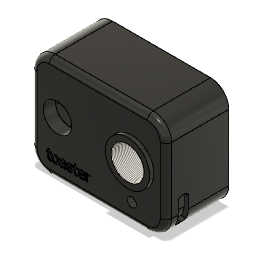
MDCEnclosure (Autodesk Fusion 360 design; units mm, degrees)
Autodesk Fusion 360 part; units mm, degrees
sketch "Board" plane through (0, 0, 0) normal (0, 0, 1) x (1, 0, 0)
  line L0 (4.75, 0) -> (39.105, 0)
  line L1 (43.855, 4.75) -> (43.855, 27.9)
  line L2 (39.105, 32.65) -> (4.75, 32.65)
  line L3 (0, 27.9) -> (0, 4.75)
  arc A0 (4.75, 32.65) -> (0, 27.9) centre (4.75, 27.9) ccw
  arc A1 (43.855, 27.9) -> (39.105, 32.65) centre (39.105, 27.9) ccw
  arc A2 (39.105, 0) -> (43.855, 4.75) centre (39.105, 4.75) ccw
  arc A3 (0, 4.75) -> (4.75, 0) centre (4.75, 4.75) ccw
  line L4 (-0.15, 27.9) -> (-0.15, 4.75)
  arc A4 (-0.15, 4.75) -> (4.75, -0.15) centre (4.75, 4.75) ccw
  line L5 (4.75, -0.15) -> (39.105, -0.15)
  arc A5 (39.105, -0.15) -> (44.005, 4.75) centre (39.105, 4.75) ccw
  line L6 (44.005, 4.75) -> (44.005, 27.9)
  arc A6 (44.005, 27.9) -> (39.105, 32.8) centre (39.105, 27.9) ccw
  line L7 (39.105, 32.8) -> (4.75, 32.8)
  arc A7 (4.75, 32.8) -> (-0.15, 27.9) centre (4.75, 27.9) ccw
  line L8 (-0.35, 27.9) -> (-0.35, 4.75)
  arc A8 (-0.35, 4.75) -> (4.75, -0.35) centre (4.75, 4.75) ccw
  line L9 (4.75, -0.35) -> (39.105, -0.35)
  arc A9 (39.105, -0.35) -> (44.205, 4.75) centre (39.105, 4.75) ccw
  line L10 (44.205, 4.75) -> (44.205, 27.9)
  arc A10 (44.205, 27.9) -> (39.105, 33) centre (39.105, 27.9) ccw
  line L11 (39.105, 33) -> (4.75, 33)
  arc A11 (4.75, 33) -> (-0.35, 27.9) centre (4.75, 27.9) ccw
  line L12 (-0.425, 27.9) -> (-0.425, 4.75)
  arc A12 (-0.425, 4.75) -> (4.75, -0.425) centre (4.75, 4.75) ccw
  line L13 (4.75, -0.425) -> (39.105, -0.425)
  arc A13 (39.105, -0.425) -> (44.28, 4.75) centre (39.105, 4.75) ccw
  line L14 (44.28, 4.75) -> (44.28, 27.9)
  arc A14 (44.28, 27.9) -> (39.105, 33.075) centre (39.105, 27.9) ccw
  line L15 (39.105, 33.075) -> (4.75, 33.075)
  arc A15 (4.75, 33.075) -> (-0.425, 27.9) centre (4.75, 27.9) ccw
  line L16 (21.9275, 32.65) -> (21.9275, 0)
  line L17 (21.9275, 33.075) -> (-21.9275, 33.075)
  line L18 (-21.9275, 33.075) -> (-21.9275, -0.425)
  line L19 (-21.9275, -0.425) -> (21.9275, -0.425)
  line L20 (21.9275, -0.425) -> (21.9275, 33.075)
  line L21 (21.9275, 33) -> (-21.9275, 33)
  line L22 (-21.9275, 33) -> (-21.9275, -0.35)
  line L23 (-21.9275, -0.35) -> (21.9275, -0.35)
  line L24 (21.9275, -0.35) -> (21.9275, 33)
  line L25 (43.855, 16.325) -> (0, 16.325)
  point P0 (21.9275, 16.325)
  dimension "d329" = 43.855
  dimension "d330" = 32.65
  dimension "d331" = 4.75
  dimension "d332" = 0.15
  dimension "d336" = 0.35
  dimension "d337" = 0.425
  dimension "d616" = 43.855
  dimension "d623" = 43.855
  dimension "d809" = 16.325
  constraint horizontal L0
  constraint vertical L1
  constraint horizontal L2
  constraint vertical L3
  constraint tangent L2 A0
  constraint tangent L3 A0
  constraint tangent L1 A1
  constraint tangent L2 A1
  constraint equal A0 A1
  constraint tangent L0 A2
  constraint tangent L1 A2
  constraint equal A0 A2
  constraint tangent L0 A3
  constraint tangent L3 A3
  constraint equal A0 A3
  constraint midpoint L2 L16.start
  constraint midpoint L0 L16.end
  constraint midpoint L16 P0
  constraint horizontal L17
  constraint vertical L18
  constraint horizontal L19
  constraint vertical L20
  constraint collinear L16 L20
  constraint collinear L13 L19
  constraint collinear L15 L17
  constraint horizontal L21
  constraint vertical L22
  constraint horizontal L23
  constraint vertical L24
  constraint collinear L16 L24
  constraint collinear L9 L23
  constraint collinear L11 L21
  constraint coincident L1 L25.start
  constraint coincident L3 L25.end
  constraint perpendicular L3 L25
  measures "d329" distance of L1 L3
  measures "d330" distance of L0 L2
  measures "d331" radius of A0
  measures "d616" distance of L18 L20
  measures "d623" distance of L22 L24
  measures "d809" distance of L0 L25
ref_plane "WorkPlane7" through (21.9275, 16.325, -3.46) normal (0, 0, 1) x (1, 0, 0)
sketch "MountPoints" plane through (0, 0, -3.46) normal (0, 0, 1) x (1, 0, 0)
  line L0 (-0.15, 27.9) -> (-0.15, 4.75)
  line L1 (4.75, -0.15) -> (39.105, -0.15)
  line L2 (3.44, 29.9) -> (0.44, 29.9)
  line L3 (0.44, 29.9) -> (0.44, 26.9)
  line L4 (0.44, 26.9) -> (3.44, 26.9)
  line L5 (3.44, 26.9) -> (3.44, 29.9)
  line L6 (3.44, 28.4) -> (0.44, 28.4)
  line L7 (0.44, 29.9) -> (-0.15, 29.9)
  line L8 (-0.15, 29.9) -> (-0.15, 26.9)
  line L9 (-0.15, 26.9) -> (0.44, 26.9)
  line L10 (0.44, 26.9) -> (0.44, 29.9)
  line L11 (3.182, 9.672) -> (0.182, 9.672)
  line L12 (0.182, 9.672) -> (0.182, 6.672)
  line L13 (0.182, 6.672) -> (3.182, 6.672)
  line L14 (3.182, 6.672) -> (3.182, 9.672)
  line L15 (3.182, 8.172) -> (0.182, 8.172)
  line L16 (0.182, 9.672) -> (-0.15, 9.672)
  line L17 (-0.15, 9.672) -> (-0.15, 6.672)
  line L18 (-0.15, 6.672) -> (0.182, 6.672)
  line L19 (0.182, 6.672) -> (0.182, 9.672)
  line L20 (44.4, 20.5) -> (39.4, 20.5)
  line L21 (39.4, 20.5) -> (39.4, 17.5)
  line L22 (39.4, 17.5) -> (44.4, 17.5)
  line L23 (44.4, 17.5) -> (44.4, 20.5)
  line L24 (44.4, 19) -> (39.4, 19)
  line L25 (44.005, 20.5) -> (44.4, 20.5)
  line L26 (44.4, 20.5) -> (44.4, 17.5)
  line L27 (44.4, 17.5) -> (44.005, 17.5)
  line L28 (44.005, 17.5) -> (44.005, 20.5)
  line L29 (44.005, 4.75) -> (44.005, 27.9)
  line L30 (0, 27.9) -> (0, 4.75)
  line L31 (4.75, 0) -> (39.105, 0)
  point P0 (1.94, 28.4)
  point P1 (1.682, 8.172)
  point P2 (41.9, 19)
  dimension "d662" = 3
  dimension "d663" = 3
  dimension "d664" = 3
  dimension "d665" = 3
  dimension "d666" = 3
  dimension "d667" = 5
  dimension "d668" = 1.682
  dimension "d669" = 8.172
  dimension "d670" = 1.94
  dimension "d671" = 28.4
  dimension "d672" = 19
  dimension "d673" = 41.9
  constraint horizontal L2
  constraint vertical L3
  constraint horizontal L4
  constraint vertical L5
  constraint midpoint L5 L6.start
  constraint midpoint L3 L6.end
  constraint midpoint P0 L6
  constraint horizontal L7
  constraint vertical L8
  constraint horizontal L9
  constraint vertical L10
  constraint collinear L0 L8
  constraint collinear L3 L10
  constraint collinear L2 L7
  constraint collinear L4 L9
  constraint horizontal L11
  constraint vertical L12
  constraint horizontal L13
  constraint vertical L14
  constraint midpoint L14 L15.start
  constraint midpoint L12 L15.end
  constraint midpoint P1 L15
  constraint horizontal L16
  constraint vertical L17
  constraint horizontal L18
  constraint vertical L19
  constraint collinear L0 L17
  constraint collinear L12 L19
  constraint collinear L11 L16
  constraint collinear L13 L18
  constraint horizontal L20
  constraint vertical L21
  constraint horizontal L22
  constraint vertical L23
  constraint midpoint L23 L24.start
  constraint midpoint L21 L24.end
  constraint midpoint P2 L24
  constraint horizontal L25
  constraint vertical L26
  constraint horizontal L27
  constraint vertical L28
  constraint collinear L28 L29
  constraint collinear L23 L26
  constraint collinear L20 L25
  constraint collinear L22 L27
  measures "d662" distance of L2 L4
  measures "d663" distance of L3 L5
  measures "d664" distance of L12 L14
  measures "d665" distance of L11 L13
  measures "d666" distance of L20 L22
  measures "d667" distance of L21 L23
  measures "d668" distance of P1 L30
  measures "d669" distance of P1 L31
  measures "d670" distance of P0 L30
  measures "d671" distance of P0 L31
  measures "d672" distance of P2 L31
  measures "d673" distance of P2 L30
sketch "BackplateMountPoints" plane through (0, 0, 0) normal (0, 0, 1) x (1, 0, 0)
  line L0 (44.005, 17.825) -> (42.505, 17.825)
  line L1 (42.505, 17.825) -> (42.505, 14.825)
  line L2 (42.505, 14.825) -> (44.005, 14.825)
  line L3 (44.005, 14.825) -> (44.005, 17.825)
  line L4 (44.005, 4.75) -> (44.005, 27.9)
  line L5 (4.75, 0) -> (39.105, 0)
  line L6 (1.35, 17.825) -> (-0.15, 17.825)
  line L7 (-0.15, 17.825) -> (-0.15, 14.825)
  line L8 (-0.15, 14.825) -> (1.35, 14.825)
  line L9 (1.35, 14.825) -> (1.35, 17.825)
  line L10 (-0.15, 27.9) -> (-0.15, 4.75)
  line L11 (44.005, 17.825) -> (44.005, 14.825)
  line L12 (-0.15, 17.825) -> (-0.15, 14.825)
  point P0 (42.505, 16.325)
  point P1 (1.35, 16.325)
  point P2 (44.005, 16.325)
  point P3 (-0.15, 16.325)
  dimension "d812" = 1.5
  dimension "d813" = 3
  dimension "d814" = 16.325
  dimension "d819" = 1.5
  dimension "d820" = 3
  dimension "d821" = 16.325
  dimension "d825" = 0
  dimension "d826" = 0
  constraint horizontal L0
  constraint vertical L1
  constraint horizontal L2
  constraint vertical L3
  constraint midpoint L1 P0
  constraint horizontal L6
  constraint vertical L7
  constraint horizontal L8
  constraint vertical L9
  constraint midpoint L9 P1
  constraint coincident L0 L3.end
  constraint coincident L2 L3.start
  constraint perpendicular L2 L11
  constraint midpoint L11 P2
  constraint collinear L3 L4
  constraint coincident L6 L7.start
  constraint coincident L8 L7.end
  constraint perpendicular L8 L12
  constraint midpoint L12 P3
  constraint collinear L7 L10
  measures "d812" distance of L1 L3
  measures "d813" distance of L0 L2
  measures "d814" distance of P0 L5
  measures "d819" distance of L7 L9
  measures "d820" distance of L6 L8
  measures "d821" distance of L5 P1
  measures "d825" distance of L3 L11
  measures "d826" distance of L7 L12
extrude "Front-Sidewalls" add sketch "Board" along normal blind 22.06 thin wall 1.5 on the left open curves L4 A4 L5 A5 L6 A6 L7 A7 makes body 1 in component "Front"
sketch "FrontHoles" plane through (0, 0, 0) normal (0, 0, 1) x (1, 0, 0)
  line L0 (0, 27.9) -> (0, 4.75)
  line L1 (4.75, 0) -> (39.105, 0)
  circle A0 centre (33.5424, 17.392) radius 7.5144
  circle A1 centre (33.5424, 17.392) radius 7.7644
  circle A2 centre (33.5424, 17.392) radius 6.8
  point P0 (7.5, 17.392)
  point P1 (33.5424, 17.392)
  point P2 (33.5424, 28.8)
  point P3 (33.5424, 4.75)
  dimension "d350" = 7.5
  dimension "d351" = 17.392
  dimension "d352" = 33.5424
  dimension "d353" = 17.392
  dimension "d554" = 15.0287
  dimension "d555" = 15.5287
  dimension "d575" = 13.6
  dimension "d647" = 33.5424
  dimension "d648" = 28.8
  dimension "d763" = 4.75
  dimension "d764" = 33.5424
  constraint coincident P1 A0.centre
  measures "d350" distance of P0 L0
  measures "d351" distance of P0 L1
  measures "d352" distance of P1 L0
  measures "d353" distance of P1 L1
  measures "d554" diameter of A0
  measures "d555" diameter of A1
  measures "d575" diameter of A2
  measures "d647" distance of L0 P2
  measures "d648" distance of L1 P2
  measures "d763" distance of L1 P3
  measures "d764" distance of L0 P3
sketch "Button" plane through (0, 0, 0) normal (0, 0, 1) x (1, 0, 0)
  circle A0 centre (33.5424, 4.75) radius 1.5
  circle A1 centre (33.5424, 4.75) radius 1.6
  circle A2 centre (33.5424, 4.75) radius 1.8
  point P0 (33.5424, 4.75)
  point P1 (33.5424, 4.75)
  dimension "d774" = 3
  dimension "d790" = 3.2
  dimension "d794" = 3.6
  constraint coincident P0 A0.centre
  constraint coincident P1 P0
  measures "d774" diameter of A0
  measures "d790" diameter of A1
  measures "d794" diameter of A2
extrude "Front-Frontplate" add sketch "Board" along normal blind 4.3 separate body contours L0 L3 A3 L16 L20 L24 L25 | L0 L2 L3 A0 A3 L4 A4 L5 L7 A7 L20 L24 | L0 L1 A2 L16 L20 L24 L25 | L0 L1 L2 A1 A2 L5 A5 L6 A6 L7 L20 L24 | L2 L3 A0 L16 L20 L24 L25 | L1 L2 A1 L16 L20 L24 L25 makes body 2 in component "Front"
hole "Front-MotionSensorHole" at (7.5, 17.392, 0) direction (0, 0, 1) diameter 9.9 depth 12 tip angle 118 bodies 2 in component "Front"
extrude "Front-LensProtrusionInside" [suppressed]
extrude "Extrude12" add sketch "FrontHoles" against normal blind 3.46 contours A0 | A2 bodies 2 in component "Front"
extrude "Front-BoardMountPoints" [suppressed]
extrude "Extrude16" add sketch "MountPoints" along normal blind 3.46 contours L0 L3 L7 L8 L9 L10 | L0 L16 L17 L18 L30 | L2 L3 L5 L6 L10 | L12 L16 L18 L19 L30 | L3 L4 L5 L6 L10 | L11 L12 L14 L15 L19 | L12 L13 L14 L15 L19 | L20 L23 L24 L25 L26 L28 L29 | L20 L21 L24 L28 L29 | L22 L23 L24 L26 L27 L28 L29 | L21 L22 L24 L28 L29 bodies 2 in component "Front"
extrude "Front-LensProtrusionBoardGap" cut sketch "FrontHoles" along normal blind 0.25 from surface at -3.46 contours A0 | A2 bodies 2 in component "Front"
extrude "Extrude24" [no effect]
extrude "Extrude18" cut sketch "FrontHoles" along normal blind 0.5 from surface at -3.21 contours A2 bodies 1 2 in component "Front"
extrude "Front-LensProtrusionOutside" [suppressed]
extrude "Extrude13" add sketch "FrontHoles" along normal blind 5.74 contours A0 | A1 | A2 bodies 2 in component "Front"
hole "Hole8" at (33.5424, 17.392, -2.71) direction (0, 0, 1) diameter 11.529 depth 20 tip angle 180 bodies 2 in component "Front"
thread "Thread2" "ISO Metric profile 12.0 M12x0.5 6H" major diameter 12.0961 minor diameter 11.5287 pitch 0.5 angle 60 resizes the face on face at (34.1164, 23.1279, 0.1067) from (33.5424, 17.392, -2.21) to (33.5424, 17.392, 5.74) on bodies 2 in component "Front"
hole "Hole10" at (1.94, 28.4, -3.46) at (1.682, 8.172, -3.46) at (41.9, 19, -3.46) direction (0, 0, 1) diameter 1.271 depth 5 tip angle 180 bodies 1 2 in component "Front"
thread "Thread4" "ISO Metric profile 1.6 M1.6x0.35 6H" major diameter 1.668 minor diameter 1.271 pitch 0.35 angle 60 resizes the face on face at (1.3283, 28.5721, -1.7933) on face at (1.7137, 8.8067, -1.7933) on face at (41.8683, 19.6347, -0.1267) on bodies 2 in component "Front"
hole "LEDHole" [suppressed] in component "Front"
hole "Hole12" at (33.5424, 4.75, 0) at (33.5424, 4.75, 0) direction (0, 0, 1) diameter 3.2 depth 4.3 tip angle 180 bodies 2 in component "Front"
move_body "MoveToFront" bodies 2 to x (1, 0, 0) y (0, 1, 0) z (0, 0, 1) at (0, 0, 17.76) in component "Front"
extrude "Extrude25" add sketch "BackplateMountPoints" along normal blind 22.06 separate body makes body 3 at (44.005, 15.825, 7.3533) makes body 4 at (-0.15, 16.825, 7.3533) in component "Front"
combine "Front-Combine" operation add target body 1 tool bodies 2 3 4 in component "Front"
hole "Hole13" at (44.005, 16.325, 0) at (-0.15, 16.325, 0) direction (0, 0, 1) diameter 1.271 depth 5 tip angle 180 bodies 1 in component "Front"
thread "Thread5" "ISO Metric profile 1.6 M1.6x0.35 6H" major diameter 1.668 minor diameter 1.271 pitch 0.35 angle 60 resizes the face on face at (43.9733, 16.9597, 3.3333) on face at (-0.7617, 16.4971, 1.6667) on bodies 1 in component "Front"
sketch "ToasterText" plane through (0, 0, 22.06) normal (0, 0, 1) x (1, 0, 0) in component "Front"
  line L0 (5.3531, 5.2645) -> (4.6727, 5.2645)
  line L1 (4.6727, 5.2645) -> (4.6727, 3.8018)
  spline S0 degree 3 poles (4.6727, 3.8018) (4.6727, 3.6947) (4.6959, 3.6197) (4.7423, 3.5768) knots 0 0 0 0 1 1 1 1
  spline S1 degree 3 poles (4.7423, 3.5768) (4.7888, 3.5339) (4.8691, 3.5125) (4.9834, 3.5125) knots 0 0 0 0 1 1 1 1
  spline S2 degree 3 poles (4.9834, 3.5125) (5.0977, 3.5125) (5.2281, 3.5286) (5.3746, 3.5607) knots 0 0 0 0 1 1 1 1
  line L2 (5.3746, 3.5607) -> (5.3746, 3.0839)
  spline S3 degree 3 poles (5.3746, 3.0839) (5.2031, 3.0303) (5.0263, 3.0035) (4.8441, 3.0035) knots 0 0 0 0 1 1 1 1
  spline S4 degree 3 poles (4.8441, 3.0035) (4.5798, 3.0035) (4.386, 3.0607) (4.2628, 3.175) knots 0 0 0 0 1 1 1 1
  spline S5 degree 3 poles (4.2628, 3.175) (4.1396, 3.2893) (4.078, 3.4875) (4.078, 3.7697) knots 0 0 0 0 1 1 1 1
  line L3 (4.078, 3.7697) -> (4.078, 5.2645)
  line L4 (4.078, 5.2645) -> (3.7083, 5.2645)
  line L5 (3.7083, 5.2645) -> (3.7083, 5.7521)
  line L6 (3.7083, 5.7521) -> (4.094, 5.7521)
  line L7 (4.094, 5.7521) -> (4.1369, 6.5236)
  line L8 (4.1369, 6.5236) -> (4.6727, 6.5236)
  line L9 (4.6727, 6.5236) -> (4.6727, 5.7521)
  line L10 (4.6727, 5.7521) -> (5.3531, 5.7521)
  line L11 (5.3531, 5.7521) -> (5.3531, 5.2645)
  spline S6 degree 3 poles (5.755, 5.452) (5.9693, 5.6949) (6.2872, 5.8164) (6.7086, 5.8164) knots 0 0 0 0 1 1 1 1
  spline S7 degree 3 poles (6.7086, 5.8164) (7.1301, 5.8164) (7.4471, 5.6949) (7.6597, 5.452) knots 0 0 0 0 1 1 1 1
  spline S8 degree 3 poles (7.6597, 5.452) (7.8722, 5.2091) (7.9784, 4.8609) (7.9784, 4.4073) knots 0 0 0 0 1 1 1 1
  line L12 (7.9784, 4.4073) -> (7.9784, 4.3965)
  spline S9 degree 3 poles (7.9784, 4.3965) (7.9784, 3.9429) (7.8722, 3.5938) (7.6597, 3.3491) knots 0 0 0 0 1 1 1 1
  spline S10 degree 3 poles (7.6597, 3.3491) (7.4471, 3.1044) (7.1301, 2.9821) (6.7086, 2.9821) knots 0 0 0 0 1 1 1 1
  spline S11 degree 3 poles (6.7086, 2.9821) (6.2872, 2.9821) (5.9702, 3.1044) (5.7576, 3.3491) knots 0 0 0 0 1 1 1 1
  spline S12 degree 3 poles (5.7576, 3.3491) (5.5451, 3.5938) (5.4388, 3.9429) (5.4388, 4.3965) knots 0 0 0 0 1 1 1 1
  line L13 (5.4388, 4.3965) -> (5.4388, 4.4073)
  spline S13 degree 3 poles (5.4388, 4.4073) (5.4388, 4.8609) (5.5442, 5.2091) (5.755, 5.452) knots 0 0 0 0 1 1 1 1
  spline S14 degree 3 poles (6.7086, 3.4803) (7.1551, 3.4803) (7.3784, 3.7857) (7.3784, 4.3965) knots 0 0 0 0 1 1 1 1
  line L14 (7.3784, 4.3965) -> (7.3784, 4.4073)
  spline S15 degree 3 poles (7.3784, 4.4073) (7.3784, 5.0145) (7.1551, 5.3181) (6.7086, 5.3181) knots 0 0 0 0 1 1 1 1
  spline S16 degree 3 poles (6.7086, 5.3181) (6.2657, 5.3181) (6.0443, 5.0145) (6.0443, 4.4073) knots 0 0 0 0 1 1 1 1
  line L15 (6.0443, 4.4073) -> (6.0443, 4.3965)
  spline S17 degree 3 poles (6.0443, 4.3965) (6.0443, 3.7857) (6.2657, 3.4803) (6.7086, 3.4803) knots 0 0 0 0 1 1 1 1
  line L16 (9.8751, 4.0911) -> (9.8751, 4.3055)
  line L17 (9.8751, 4.3055) -> (9.4143, 4.2626)
  spline S18 degree 3 poles (9.4143, 4.2626) (9.1536, 4.2376) (8.9661, 4.1956) (8.8518, 4.1367) knots 0 0 0 0 1 1 1 1
  spline S19 degree 3 poles (8.8518, 4.1367) (8.7375, 4.0777) (8.6803, 3.9697) (8.6803, 3.8125) knots 0 0 0 0 1 1 1 1
  line L18 (8.6803, 3.8125) -> (8.6803, 3.8018)
  spline S20 degree 3 poles (8.6803, 3.8018) (8.6803, 3.6875) (8.7169, 3.6) (8.7902, 3.5393) knots 0 0 0 0 1 1 1 1
  spline S21 degree 3 poles (8.7902, 3.5393) (8.8634, 3.4786) (8.9643, 3.4482) (9.0929, 3.4482) knots 0 0 0 0 1 1 1 1
  spline S22 degree 3 poles (9.0929, 3.4482) (9.3286, 3.4482) (9.5179, 3.5098) (9.6608, 3.633) knots 0 0 0 0 1 1 1 1
  spline S23 degree 3 poles (9.6608, 3.633) (9.8037, 3.7563) (9.8751, 3.909) (9.8751, 4.0911) knots 0 0 0 0 1 1 1 1
  line L19 (8.8196, 4.943) -> (8.2356, 4.943)
  spline S24 degree 3 poles (8.2356, 4.943) (8.2463, 5.2181) (8.3472, 5.4315) (8.5383, 5.5833) knots 0 0 0 0 1 1 1 1
  spline S25 degree 3 poles (8.5383, 5.5833) (8.7294, 5.7351) (9.0125, 5.811) (9.3876, 5.811) knots 0 0 0 0 1 1 1 1
  spline S26 degree 3 poles (9.3876, 5.811) (10.1019, 5.811) (10.4591, 5.511) (10.4591, 4.9109) knots 0 0 0 0 1 1 1 1
  line L20 (10.4591, 4.9109) -> (10.4591, 3.0517)
  line L21 (10.4591, 3.0517) -> (9.918, 3.0517)
  line L22 (9.918, 3.0517) -> (9.9019, 3.4321)
  line L23 (9.9019, 3.4321) -> (9.8912, 3.4321)
  spline S27 degree 3 poles (9.8912, 3.4321) (9.8162, 3.3) (9.6992, 3.1928) (9.5403, 3.1107) knots 0 0 0 0 1 1 1 1
  spline S28 degree 3 poles (9.5403, 3.1107) (9.3813, 3.0285) (9.1982, 2.9874) (8.9911, 2.9874) knots 0 0 0 0 1 1 1 1
  spline S29 degree 3 poles (8.9911, 2.9874) (8.7196, 2.9874) (8.5026, 3.0517) (8.3401, 3.1803) knots 0 0 0 0 1 1 1 1
  spline S30 degree 3 poles (8.3401, 3.1803) (8.1776, 3.3089) (8.0963, 3.5054) (8.0963, 3.7697) knots 0 0 0 0 1 1 1 1
  line L24 (8.0963, 3.7697) -> (8.0963, 3.7804)
  spline S31 degree 3 poles (8.0963, 3.7804) (8.0963, 3.9161) (8.1186, 4.034) (8.1633, 4.134) knots 0 0 0 0 1 1 1 1
  spline S32 degree 3 poles (8.1633, 4.134) (8.2079, 4.234) (8.266, 4.3144) (8.3374, 4.3751) knots 0 0 0 0 1 1 1 1
  spline S33 degree 3 poles (8.3374, 4.3751) (8.4089, 4.4358) (8.5017, 4.4858) (8.616, 4.5251) knots 0 0 0 0 1 1 1 1
  spline S34 degree 3 poles (8.616, 4.5251) (8.7303, 4.5644) (8.8411, 4.593) (8.9482, 4.6108) knots 0 0 0 0 1 1 1 1
  spline S35 degree 3 poles (8.9482, 4.6108) (9.0554, 4.6287) (9.184, 4.6448) (9.334, 4.6591) knots 0 0 0 0 1 1 1 1
  line L25 (9.334, 4.6591) -> (9.8698, 4.7073)
  line L26 (9.8698, 4.7073) -> (9.8698, 4.9109)
  spline S36 degree 3 poles (9.8698, 4.9109) (9.8698, 5.0538) (9.834, 5.16) (9.7626, 5.2297) knots 0 0 0 0 1 1 1 1
  spline S37 degree 3 poles (9.7626, 5.2297) (9.6912, 5.2993) (9.5661, 5.3342) (9.3876, 5.3342) knots 0 0 0 0 1 1 1 1
  spline S38 degree 3 poles (9.3876, 5.3342) (9.0232, 5.3342) (8.8339, 5.2038) (8.8196, 4.943) knots 0 0 0 0 1 1 1 1
  spline S39 degree 3 poles (11.8629, 3.4589) (12.2201, 3.4589) (12.3986, 3.575) (12.3986, 3.8072) knots 0 0 0 0 1 1 1 1
  line L27 (12.3986, 3.8072) -> (12.3986, 3.8179)
  spline S40 degree 3 poles (12.3986, 3.8179) (12.3986, 3.9179) (12.3594, 3.9947) (12.2808, 4.0483) knots 0 0 0 0 1 1 1 1
  spline S41 degree 3 poles (12.2808, 4.0483) (12.2022, 4.1019) (12.0807, 4.1394) (11.9164, 4.1608) knots 0 0 0 0 1 1 1 1
  line L28 (11.9164, 4.1608) -> (11.6539, 4.1929)
  spline S42 degree 3 poles (11.6539, 4.1929) (11.3432, 4.2287) (11.1101, 4.3081) (10.9547, 4.4314) knots 0 0 0 0 1 1 1 1
  spline S43 degree 3 poles (10.9547, 4.4314) (10.7993, 4.5546) (10.7216, 4.7484) (10.7216, 5.0127) knots 0 0 0 0 1 1 1 1
  line L29 (10.7216, 5.0127) -> (10.7216, 5.0234)
  spline S44 degree 3 poles (10.7216, 5.0234) (10.7216, 5.2806) (10.8136, 5.477) (10.9976, 5.6128) knots 0 0 0 0 1 1 1 1
  spline S45 degree 3 poles (10.9976, 5.6128) (11.1815, 5.7485) (11.4539, 5.8164) (11.8146, 5.8164) knots 0 0 0 0 1 1 1 1
  spline S46 degree 3 poles (11.8146, 5.8164) (12.5183, 5.8164) (12.888, 5.5431) (12.9237, 4.9966) knots 0 0 0 0 1 1 1 1
  line L30 (12.9237, 4.9966) -> (12.3451, 4.9966)
  spline S47 degree 3 poles (12.3451, 4.9966) (12.3379, 5.1216) (12.2915, 5.2109) (12.2058, 5.2645) knots 0 0 0 0 1 1 1 1
  spline S48 degree 3 poles (12.2058, 5.2645) (12.12, 5.3181) (11.9897, 5.3449) (11.8146, 5.3449) knots 0 0 0 0 1 1 1 1
  spline S49 degree 3 poles (11.8146, 5.3449) (11.4717, 5.3449) (11.3003, 5.2413) (11.3003, 5.0341) knots 0 0 0 0 1 1 1 1
  line L31 (11.3003, 5.0341) -> (11.3003, 5.0234)
  spline S50 degree 3 poles (11.3003, 5.0234) (11.3003, 4.9234) (11.3396, 4.8475) (11.4182, 4.7957) knots 0 0 0 0 1 1 1 1
  spline S51 degree 3 poles (11.4182, 4.7957) (11.4967, 4.7439) (11.6253, 4.7073) (11.8039, 4.6859) knots 0 0 0 0 1 1 1 1
  line L32 (11.8039, 4.6859) -> (12.0504, 4.6537)
  spline S52 degree 3 poles (12.0504, 4.6537) (12.3719, 4.6073) (12.6067, 4.5224) (12.7549, 4.3992) knots 0 0 0 0 1 1 1 1
  spline S53 degree 3 poles (12.7549, 4.3992) (12.9032, 4.276) (12.9773, 4.0804) (12.9773, 3.8125) knots 0 0 0 0 1 1 1 1
  line L33 (12.9773, 3.8125) -> (12.9773, 3.8018)
  spline S54 degree 3 poles (12.9773, 3.8018) (12.9773, 3.2553) (12.6005, 2.9821) (11.8468, 2.9821) knots 0 0 0 0 1 1 1 1
  spline S55 degree 3 poles (11.8468, 2.9821) (11.0645, 2.9821) (10.6663, 3.2785) (10.652, 3.8715) knots 0 0 0 0 1 1 1 1
  line L34 (10.652, 3.8715) -> (11.236, 3.8715)
  spline S56 degree 3 poles (11.236, 3.8715) (11.2431, 3.7357) (11.303, 3.633) (11.4155, 3.5634) knots 0 0 0 0 1 1 1 1
  spline S57 degree 3 poles (11.4155, 3.5634) (11.528, 3.4937) (11.6771, 3.4589) (11.8629, 3.4589) knots 0 0 0 0 1 1 1 1
  line L35 (14.6811, 5.2645) -> (14.0006, 5.2645)
  line L36 (14.0006, 5.2645) -> (14.0006, 3.8018)
  spline S58 degree 3 poles (14.0006, 3.8018) (14.0006, 3.6947) (14.0238, 3.6197) (14.0703, 3.5768) knots 0 0 0 0 1 1 1 1
  spline S59 degree 3 poles (14.0703, 3.5768) (14.1167, 3.5339) (14.1971, 3.5125) (14.3114, 3.5125) knots 0 0 0 0 1 1 1 1
  spline S60 degree 3 poles (14.3114, 3.5125) (14.4257, 3.5125) (14.5561, 3.5286) (14.7025, 3.5607) knots 0 0 0 0 1 1 1 1
  line L37 (14.7025, 3.5607) -> (14.7025, 3.0839)
  spline S61 degree 3 poles (14.7025, 3.0839) (14.5311, 3.0303) (14.3542, 3.0035) (14.1721, 3.0035) knots 0 0 0 0 1 1 1 1
  spline S62 degree 3 poles (14.1721, 3.0035) (13.9078, 3.0035) (13.714, 3.0607) (13.5908, 3.175) knots 0 0 0 0 1 1 1 1
  spline S63 degree 3 poles (13.5908, 3.175) (13.4675, 3.2893) (13.4059, 3.4875) (13.4059, 3.7697) knots 0 0 0 0 1 1 1 1
  line L38 (13.4059, 3.7697) -> (13.4059, 5.2645)
  line L39 (13.4059, 5.2645) -> (13.0362, 5.2645)
  line L40 (13.0362, 5.2645) -> (13.0362, 5.7521)
  line L41 (13.0362, 5.7521) -> (13.422, 5.7521)
  line L42 (13.422, 5.7521) -> (13.4648, 6.5236)
  line L43 (13.4648, 6.5236) -> (14.0006, 6.5236)
  line L44 (14.0006, 6.5236) -> (14.0006, 5.7521)
  line L45 (14.0006, 5.7521) -> (14.6811, 5.7521)
  line L46 (14.6811, 5.7521) -> (14.6811, 5.2645)
  spline S64 degree 3 poles (16.2134, 3.4696) (16.4706, 3.4696) (16.7563, 3.525) (17.0707, 3.6357) knots 0 0 0 0 1 1 1 1
  line L47 (17.0707, 3.6357) -> (17.0707, 3.1535)
  spline S65 degree 3 poles (17.0707, 3.1535) (16.792, 3.0392) (16.492, 2.9821) (16.1705, 2.9821) knots 0 0 0 0 1 1 1 1
  spline S66 degree 3 poles (16.1705, 2.9821) (15.6812, 2.9821) (15.324, 3.0999) (15.099, 3.3357) knots 0 0 0 0 1 1 1 1
  spline S67 degree 3 poles (15.099, 3.3357) (14.874, 3.5714) (14.7614, 3.925) (14.7614, 4.3965) knots 0 0 0 0 1 1 1 1
  line L48 (14.7614, 4.3965) -> (14.7614, 4.4073)
  spline S68 degree 3 poles (14.7614, 4.4073) (14.7614, 4.8573) (14.8704, 5.2047) (15.0883, 5.4493) knots 0 0 0 0 1 1 1 1
  spline S69 degree 3 poles (15.0883, 5.4493) (15.3062, 5.694) (15.624, 5.8164) (16.042, 5.8164) knots 0 0 0 0 1 1 1 1
  spline S70 degree 3 poles (16.042, 5.8164) (16.8206, 5.8164) (17.21, 5.3895) (17.21, 4.5358) knots 0 0 0 0 1 1 1 1
  spline S71 degree 3 poles (17.21, 4.5358) (17.21, 4.4358) (17.1992, 4.318) (17.1778, 4.1822) knots 0 0 0 0 1 1 1 1
  line L49 (17.1778, 4.1822) -> (15.3401, 4.1822)
  spline S72 degree 3 poles (15.3401, 4.1822) (15.3472, 3.9358) (15.4196, 3.7554) (15.5571, 3.6411) knots 0 0 0 0 1 1 1 1
  spline S73 degree 3 poles (15.5571, 3.6411) (15.6946, 3.5268) (15.9134, 3.4696) (16.2134, 3.4696) knots 0 0 0 0 1 1 1 1
  spline S74 degree 3 poles (16.5081, 5.1627) (16.4188, 5.2841) (16.2616, 5.3449) (16.0366, 5.3449) knots 0 0 0 0 1 1 1 1
  spline S75 degree 3 poles (16.0366, 5.3449) (15.8116, 5.3449) (15.6437, 5.285) (15.533, 5.1654) knots 0 0 0 0 1 1 1 1
  spline S76 degree 3 poles (15.533, 5.1654) (15.4222, 5.0457) (15.3579, 4.8609) (15.3401, 4.6108) knots 0 0 0 0 1 1 1 1
  line L50 (15.3401, 4.6108) -> (16.6474, 4.6108)
  spline S77 degree 3 poles (16.6474, 4.6108) (16.6438, 4.8609) (16.5974, 5.0448) (16.5081, 5.1627) knots 0 0 0 0 1 1 1 1
  line L51 (17.4457, 3.0517) -> (17.4457, 5.7521)
  line L52 (17.4457, 5.7521) -> (18.0297, 5.7521)
  line L53 (18.0297, 5.7521) -> (18.0404, 5.2538)
  line L54 (18.0404, 5.2538) -> (18.0511, 5.2538)
  spline S78 degree 3 poles (18.0511, 5.2538) (18.1047, 5.4181) (18.202, 5.5556) (18.3431, 5.6663) knots 0 0 0 0 1 1 1 1
  spline S79 degree 3 poles (18.3431, 5.6663) (18.4842, 5.7771) (18.678, 5.8235) (18.9245, 5.8056) knots 0 0 0 0 1 1 1 1
  line L55 (18.9245, 5.8056) -> (18.9245, 5.2163)
  spline S80 degree 3 poles (18.9245, 5.2163) (18.6101, 5.2163) (18.3842, 5.1511) (18.2467, 5.0207) knots 0 0 0 0 1 1 1 1
  spline S81 degree 3 poles (18.2467, 5.0207) (18.1092, 4.8903) (18.0404, 4.6751) (18.0404, 4.3751) knots 0 0 0 0 1 1 1 1
  line L56 (18.0404, 4.3751) -> (18.0404, 3.0517)
  line L57 (18.0404, 3.0517) -> (17.4457, 3.0517)
  circle A0 centre (33.5424, 17.392) radius 7.7643
  line L58 (-1.65, 27.9) -> (-1.65, 4.75)
  arc A1 (-1.65, 4.75) -> (4.75, -1.65) centre (4.75, 4.75) ccw
  line L59 (4.75, -1.65) -> (39.105, -1.65)
  arc A2 (39.105, -1.65) -> (45.505, 4.75) centre (39.105, 4.75) ccw
  line L60 (45.505, 4.75) -> (45.505, 27.9)
  arc A3 (45.505, 27.9) -> (39.105, 34.3) centre (39.105, 27.9) ccw
  line L61 (39.105, 34.3) -> (4.75, 34.3)
  arc A4 (4.75, 34.3) -> (-1.65, 27.9) centre (4.75, 27.9) ccw
  circle A5 centre (33.5424, 4.75) radius 1.6
  circle A6 centre (7.5, 17.392) radius 4.95
extrude "ToasterTextExtrude" cut sketch "ToasterText" against normal blind 0.25 contours L0 L1 S0 S1 S2 L2 S3 S4 S5 L3 L4 L5 L6 L7 L8 L9 L10 L11 | S6 S7 S8 L12 S9 S10 S11 S12 L13 S13 | L19 S24 S25 S26 L20 L21 L22 L23 S27 S28 S29 S30 L24 S31 S32 S33 S34 S35 L25 L26 S36 S37 S38 | S39 L27 S40 S41 L28 S42 S43 L29 S44 S45 S46 L30 S47 S48 S49 L31 S50 S51 L32 S52 S53 L33 S54 S55 L34 S56 S57 | L35 L36 S58 S59 S60 L37 S61 S62 S63 L38 L39 L40 L41 L42 L43 L44 L45 L46 | S64 L47 S65 S66 S67 L48 S68 S69 S70 S71 L49 S72 S73 | L51 L52 L53 L54 S78 S79 L55 S80 S81 L56 L57 bodies 1 in component "Front"
fillet "Fillet Text Corners" radius 0.1 33 edges at (4.1369, 6.5236, 21.935) (4.6727, 6.5236, 21.935) (3.7083, 5.7521, 21.935) (3.7083, 5.2645, 21.935) (5.3531, 5.7521, 21.935) (5.3531, 5.2645, 21.935) (5.3746, 3.5607, 21.935) (5.3746, 3.0839, 21.935) (8.2356, 4.943, 21.935) (8.8196, 4.943, 21.935) (9.918, 3.0517, 21.935) (10.4591, 3.0517, 21.935) (10.652, 3.8715, 21.935) (11.236, 3.8715, 21.935) (12.3451, 4.9966, 21.935) (12.9237, 4.9966, 21.935) (13.4648, 6.5236, 21.935) (14.0006, 6.5236, 21.935) (13.0362, 5.7521, 21.935) (13.0362, 5.2645, 21.935) (14.6811, 5.7521, 21.935) (14.6811, 5.2645, 21.935) (14.7025, 3.5607, 21.935) (14.7025, 3.0839, 21.935) (17.1778, 4.1822, 21.935) (17.0707, 3.6357, 21.935) (17.0707, 3.1535, 21.935) (17.4457, 5.7521, 21.935) (18.0297, 5.7521, 21.935) (17.4457, 3.0517, 21.935) (18.0404, 3.0517, 21.935) (18.9245, 5.8056, 21.935) (18.9245, 5.2163, 21.935) on bodies 1 in component "Front"
fillet "Fillet4" radius 1.5 8 edges at (3.44, 29.9, 16.03) (3.44, 26.9, 16.03) (3.182, 9.672, 16.03) (3.182, 6.672, 16.03) (42.505, 17.825, 7.15) (42.505, 14.825, 8.88) (1.35, 17.825, 8.88) (1.35, 14.825, 8.88) on bodies 1 in component "Front"
fillet "Fillet5" radius 1 9 edges at (-0.15, 26.9, 16.03) (0.2767, 29.9, 16.03) (44.005, 20.5, 16.03) (-0.15, 9.672, 16.03) (-0.15, 6.672, 16.03) (-0.15, 17.825, 8.88) (-0.15, 14.825, 8.88) (44.005, 17.825, 7.15) (44.005, 14.825, 8.88) on bodies 1 in component "Front"
fillet "Fillet16" radius 1 1 edges at (40.3839, 20.5, 16.155) on bodies 1 in component "Front"
fillet "Fillet17" radius 0.75 1 edges at (41.056, 17.5, 16.155) on bodies 1 in component "Front"
fillet "Fillet18" radius 0.75 1 edges at (43.0726, 17.5, 16.03) on bodies 1 in component "Front"
fillet "Fillet19" radius 1 2 edges at (40.3839, 20.5, 14.425) (41.056, 17.5, 14.425) on bodies 1 in component "Front"
fillet "FrontFillet" radius 2 8 edges at (-1.65, 16.325, 22.06) (0.2245, 0.2245, 22.06) (21.9275, -1.65, 22.06) (43.6305, 0.2245, 22.06) (45.505, 16.325, 22.06) (43.6305, 32.4255, 22.06) (21.9275, 34.3, 22.06) (0.2245, 32.4255, 22.06) on bodies 1 in component "Front"
extrude "Extrude1" add sketch "Button" along normal blind 7.66 separate body contours A0 makes body 5 in component "Button"
extrude "Extrude2" add sketch "Button" along normal blind 2.76 contours A0 | A1 | A2 bodies 5 in component "Button"
move_body "Align1" bodies 5 to x (1, 0, 0) y (0, 1, 0) z (0, 0, 1) at (0, 0, 14.4) in component "Button"
move_body "Move1" bodies 5 to x (1, 0, 0) y (0, 1, 0) z (0, 0, 1) at (0, 0, 0.6) in component "Button"
sketch "USBCPlugCutout" plane through (0, 0, 0) normal (1, 0, 0) x (0, 0, -1) in component "Front"
  line L0 (-22, 4.75) -> (-22, 27.9)
  line L1 (-22, 27.9) -> (-23.5, 27.9)
  line L2 (-23.5, 27.9) -> (-23.5, 4.75)
  line L3 (-23.5, 4.75) -> (-22, 4.75)
  line L4 (-18.715, 19.0109) -> (-17.155, 19.0109)
  line L5 (-16.155, 18.0109) -> (-16.155, 10.6709)
  line L6 (-17.155, 9.6709) -> (-18.715, 9.6709)
  line L7 (-19.715, 10.6709) -> (-19.715, 18.0109)
  arc A0 (-18.715, 19.0109) -> (-19.715, 18.0109) centre (-18.715, 18.0109) ccw
  arc A1 (-16.155, 18.0109) -> (-17.155, 19.0109) centre (-17.155, 18.0109) ccw
  arc A2 (-17.155, 9.6709) -> (-16.155, 10.6709) centre (-17.155, 10.6709) ccw
  arc A3 (-19.715, 10.6709) -> (-18.715, 9.6709) centre (-18.715, 10.6709) ccw
  dimension "d492" = 3.56
  dimension "d493" = 9.34
  dimension "d497" = 1
  dimension "d498" = 1
  dimension "d499" = 1
  constraint horizontal L4
  constraint vertical L5
  constraint vertical L7
  constraint tangent L4 A0
  constraint tangent L7 A0
  constraint tangent L4 A1
  constraint tangent L5 A1
  constraint tangent L5 A2
  constraint tangent L6 A2
  constraint tangent L6 A3
  constraint tangent L7 A3
  constraint equal A2 A3
  measures "d492" distance of L5 L7
  measures "d493" distance of L4 L6
  measures "d497" radius of A0
  measures "d498" radius of A1
  measures "d499" radius of A2
extrude "Extrude9" add sketch "USBCPlugCutout" along normal blind 10 separate body contours L4 L5 L6 L7 A0 A1 A2 A3 makes body 6 in component "Front"
ref_plane "WorkPlane5" through (42.1944, 19, 14.2) normal (0, 0, -1) x (-1, 0, 0) in component "Front"
ref_plane "WorkPlane6" through (42.005, 16.325, 11.03) normal (-1, 0, 0) x (0, -1, 0) in component "Front"
move_body "Align3" bodies 6 to x (1, 0, 0) y (0, 1, 0) z (0, 0, 1) at (42.005, 0, 0) in component "Front"
move_body "Align4" bodies 6 to x (1, 0, 0) y (0, 1, 0) z (0, 0, 1) at (0, 0, -1.955) in component "Front"
ref_plane "WorkPlane7" through (21.9275, 0, 0) normal (0, -1, 0) x (1, 0, 0) in component "Front"
ref_plane "WorkPlane9" through (21.9275, 5.2535, 0) normal (0, -1, 0) x (1, 0, 0) in component "Front"
move_body "Align5" bodies 6 to x (1, 0, 0) y (0, 1, 0) z (0, 0, 1) at (0, -9.0874, 0) in component "Front"
combine "Combine3" operation cut target body 1 tool bodies 6 in component "Front"
extrude "Extrude7" add sketch "Board" along normal blind 1.5 thin wall 1.5 on the left separate body open curves A4 L5 A5 L6 A6 L7 A7 L4 makes body 7 in component "Backplate"
extrude "Extrude8" add sketch "Board" along normal blind 1.5 contours L0 L3 A3 L16 L20 L24 L25 | L0 L2 L3 A0 A3 L4 A4 L5 L7 A7 L20 L24 | L0 L1 A2 L16 L20 L24 L25 | L0 L1 L2 A1 A2 L5 A5 L6 A6 L7 L20 L24 | L2 L3 A0 L16 L20 L24 L25 | L1 L2 A1 L16 L20 L24 L25 bodies 7 in component "Backplate"
move_body "Align11" bodies 7 to x (1, 0, 0) y (0, 1, 0) z (0, 0, 1) at (0, 0, -1.5) in component "Backplate"
sketch "BackplateHoles" plane through (0, 0, -1.5) normal (0, 0, -1) x (-1, 0, 0) in component "Backplate"
  arc A0 (-4.75, -1.65) -> (1.65, 4.75) centre (-4.75, 4.75) ccw
  line L0 (1.65, 4.75) -> (1.65, 27.9)
  arc A1 (1.65, 27.9) -> (-4.75, 34.3) centre (-4.75, 27.9) ccw
  line L1 (-4.75, 34.3) -> (-39.105, 34.3)
  arc A2 (-39.105, 34.3) -> (-45.505, 27.9) centre (-39.105, 27.9) ccw
  line L2 (-45.505, 27.9) -> (-45.505, 4.75)
  arc A3 (-45.505, 4.75) -> (-39.105, -1.65) centre (-39.105, 4.75) ccw
  line L3 (-39.105, -1.65) -> (-4.75, -1.65)
  point P0 (-44.005, 16.325)
  point P1 (-44.005, 16.325)
  point P2 (0.15, 16.325)
  point P3 (0.15, 16.325)
  constraint coincident P1 P0
  constraint coincident P3 P2
hole "Hole2" at (44.005, 16.325, -1.5) at (-0.15, 16.325, -1.5) direction (0, 0, 1) diameter 1.271 depth 1.5 tip angle 180 countersink diameter 3 countersink angle 90 bodies 7 in component "Backplate"
sketch "Board (2)" plane through (0, 0, 0) normal (0, 0, 1) x (1, 0, 0) in component "Board"
  line L0 (4.75, 0) -> (39.105, 0)
  arc A0 (0, 4.75) -> (4.75, 0) centre (4.75, 4.75) ccw
  line L1 (0, 27.9) -> (0, 4.75)
  line L2 (41.5, 27.94) -> (41.5, 32.002)
  arc A1 (39.105, 0) -> (43.855, 4.75) centre (39.105, 4.75) ccw
  arc A2 (41.5, 32.002) -> (39.105, 32.65) centre (39.105, 27.9) ccw
  line L3 (39.105, 32.65) -> (4.75, 32.65)
  arc A3 (4.75, 32.65) -> (0, 27.9) centre (4.75, 27.9) ccw
  line L4 (43.855, 4.75) -> (43.855, 27.94)
  line L5 (41.5, 27.94) -> (43.855, 27.94)
  arc A4 (1.6764, 7.5345) -> (1.6764, 8.8095) centre (1.6764, 8.172) ccw
  arc A5 (41.9, 18.0295) -> (41.9, 16.7545) centre (41.9, 17.392) ccw
  arc A6 (41.9, 16.7545) -> (41.9, 18.0295) centre (41.9, 17.392) ccw
  arc A7 (1.6764, 8.8095) -> (1.6764, 7.5345) centre (1.6764, 8.172) ccw
  arc A8 (1.6764, 8.8095) -> (1.6764, 7.5345) centre (1.6764, 8.172) ccw
  arc A9 (41.9, 18.0295) -> (41.9, 16.7545) centre (41.9, 17.392) ccw
  arc A10 (41.9, 16.7545) -> (41.9, 18.0295) centre (41.9, 17.392) ccw
  arc A11 (41.9, 18.0295) -> (41.9, 16.7545) centre (41.9, 17.392) ccw
  arc A12 (1.94, 29.0375) -> (1.94, 27.7625) centre (1.94, 28.4) ccw
  arc A13 (1.6764, 8.8095) -> (1.6764, 7.5345) centre (1.6764, 8.172) ccw
  arc A14 (1.6764, 7.5345) -> (1.6764, 8.8095) centre (1.6764, 8.172) ccw
  arc A15 (1.94, 27.7625) -> (1.94, 29.0375) centre (1.94, 28.4) ccw
  arc A16 (1.94, 29.0375) -> (1.94, 27.7625) centre (1.94, 28.4) ccw
  arc A17 (1.6764, 8.8095) -> (1.6764, 7.5345) centre (1.6764, 8.172) ccw
  arc A18 (1.94, 27.7625) -> (1.94, 29.0375) centre (1.94, 28.4) ccw
  arc A19 (41.9, 18.0295) -> (41.9, 16.7545) centre (41.9, 17.392) ccw
  arc A20 (41.9, 16.7545) -> (41.9, 18.0295) centre (41.9, 17.392) ccw
  arc A21 (41.9, 16.7545) -> (41.9, 18.0295) centre (41.9, 17.392) ccw
  arc A22 (1.6764, 7.5345) -> (1.6764, 8.8095) centre (1.6764, 8.172) ccw
  arc A23 (1.94, 29.0375) -> (1.94, 27.7625) centre (1.94, 28.4) ccw
  arc A24 (1.94, 27.7625) -> (1.94, 29.0375) centre (1.94, 28.4) ccw
  arc A25 (1.94, 27.7625) -> (1.94, 29.0375) centre (1.94, 28.4) ccw
  arc A26 (1.94, 29.0375) -> (1.94, 27.7625) centre (1.94, 28.4) ccw
  arc A27 (1.6764, 7.5345) -> (1.6764, 8.8095) centre (1.6764, 8.172) ccw
  arc A28 (1.94, 29.0692) -> (1.94, 27.7308) centre (1.94, 28.4) ccw
  arc A29 (1.6764, 8.8413) -> (1.6764, 7.5028) centre (1.6764, 8.172) ccw
  arc A30 (1.94, 27.7308) -> (1.94, 29.0692) centre (1.94, 28.4) ccw
  arc A31 (41.9, 18.0612) -> (41.9, 16.7228) centre (41.9, 17.392) ccw
  arc A32 (1.6764, 7.5028) -> (1.6764, 8.8413) centre (1.6764, 8.172) ccw
  arc A33 (41.9, 16.7228) -> (41.9, 18.0612) centre (41.9, 17.392) ccw
  arc A34 (1.94, 27.7308) -> (1.94, 29.0692) centre (1.94, 28.4) ccw
  arc A35 (41.9, 18.0612) -> (41.9, 16.7228) centre (41.9, 17.392) ccw
  arc A36 (1.6764, 8.8413) -> (1.6764, 7.5028) centre (1.6764, 8.172) ccw
  arc A37 (1.94, 29.0692) -> (1.94, 27.7308) centre (1.94, 28.4) ccw
  arc A38 (41.9, 16.7228) -> (41.9, 18.0612) centre (41.9, 17.392) ccw
  arc A39 (1.6764, 7.5028) -> (1.6764, 8.8413) centre (1.6764, 8.172) ccw
  point P0 (1.6764, 8.172)
  point P1 (41.9, 17.392)
  point P2 (1.94, 28.4)
extrude "Board" add sketch "Board (2)" along normal blind 3.1 separate body contours L0 A0 L1 L2 A1 A2 L3 A3 L4 L5 makes body 8 in component "Board"
move_body "Board (1)" bodies 8 to x (1, 0, 0) y (0, 1, 0) z (0, 0, 1) at (0, 0, 11.2) in component "Board"
sketch "Sketch1" plane through (0, 0, 0) normal (0, 0, 1) x (1, 0, 0) in component "Battery"
  line L0 (20, 15) -> (-20, 15)
  line L1 (-20, 15) -> (-20, -15)
  line L2 (-20, -15) -> (20, -15)
  line L3 (20, -15) -> (20, 15)
  line L4 (20, 15) -> (-20, -15) construction
  dimension "d443" = 40
  dimension "d444" = 30
  constraint horizontal L0
  constraint vertical L1
  constraint horizontal L2
  constraint vertical L3
  constraint midpoint L4 origin
  measures "d443" distance of L1 L3
  measures "d444" distance of L0 L2
extrude "Extrude1'" add sketch "Sketch1" along normal blind 11.2 separate body makes body 9 in component "Battery"
move_body "Align1'" bodies 9 to x (1, 0, 0) y (0, 1, 0) z (0, 0, 1) at (21.9275, 16.325, 0) in component "Battery"
component "Front" placed x (1, 0, 0) y (0, 1, 0) z (0, 0, 1) at (0, 0, 0)
component "Button" placed x (1, 0, 0) y (0, 1, 0) z (0, 0, 1) at (0, 0, 0)
component "Backplate" placed x (1, 0, 0) y (0, 1, 0) z (0, 0, 1) at (0, 0, 0)
component "Board" placed x (1, 0, 0) y (0, 1, 0) z (0, 0, 1) at (0, 0, 0)
component "Battery" placed x (1, 0, 0) y (0, 1, 0) z (0, 0, 1) at (0, 0, 0)
equation "BoardHeight = 32.65 mm"
equation "BoardWidth = 43.855 mm"
equation "EnclosureThickness = 1.5 mm"
equation "ImageSensorX = 33.5424 mm"
equation "ImageSensorY = 17.392 mm"
equation "MotionSensorX = 7.5 mm"
equation "MotionSensorY = 17.392 mm"
equation "MotionSensorDiameter = 9.3 mm + 0.5 mm + EnclosureMfgTol"
equation "LensProtrusionOutsideThickness = 13.5287 mm + 2 mm"
equation "LensProtrusionDepth = LensThreadDepth - MountPointDepth"
equation "OuterEdgeRadius = 6 mm"
equation "BoardRadius = 4.75 mm"
equation "MountPoint2X = 1.682 mm"
equation "MountPoint2Y = 8.172 mm"
equation "MountPointDepth = USBCReceptacleWidth + 0.3 mm"
equation "MountPoint3X = 41.9 mm"
equation "MountPoint3Y = 19 mm"
equation "MountPoint1X = 1.94 mm"
equation "MountPoint1Y = 28.4 mm"
equation "BackplateMountPointDepth = EnclosureDepth"
equation "BackplateMountPointWidth = 1.5 mm"
equation "HoleDiameter = 10 mm"
equation "BatteryWidth = 40 mm"
equation "BatteryHeight = 30 mm"
equation "BatteryThickness = 11 mm + 0.2 mm"
equation "BackplateOverlap = 0.2 mm"
equation "BackplateHoleOffset = ( BackplateMountPointWidth - EnclosureThickness ) / 2"
equation "ScrewHeadDiameter = 3 mm"
equation "ScrewHeadHeight = 1 mm"
equation "BackplateThickness = 1.5 mm"
equation "EnclosureDepth = FrontplateThickness + MountPointDepth + BoardThickness + BatteryThickness"
equation "BoardThickness = 3.1 mm"
equation "BoardEnclosureGap = 0.15 mm"
equation "USBCReceptacleCutoutWidth = USBCReceptacleWidth + USBCReceptacleTolerance + 2 * EnclosureMfgTol"
equation "USBCReceptacleCutoutHeight = USBCReceptacleHeight + USBCReceptacleTolerance + 2 * EnclosureMfgTol"
equation "USBCReceptacleCutoutRadius = 2.4 mm / 2 - 0.2 mm"
equation "USBCReceptacleY = 5.25348125 mm"
equation "USBCReceptacleWidth = 3.16 mm"
equation "d329 = BoardWidth"
equation "d330 = BoardHeight"
equation "d331 = BoardRadius"
equation "d332 = BoardEnclosureGap"
equation "d333 = EnclosureThickness"
equation "d334 = EnclosureDepth"
equation "d336 = BoardEnclosureGap + BackplateOverlap"
equation "d337 = BoardEnclosureGap + BackplateOverlap + BackplateGap"
equation "d350 = MotionSensorX"
equation "d351 = MotionSensorY"
equation "d352 = ImageSensorX"
equation "d353 = ImageSensorY"
equation "d354 = FrontplateThickness"
equation "d363 = MotionSensorDiameter"
equation "MountPointHeight = 3 mm"
equation "MountPointRadius = 1.5 mm"
equation "d443 = BatteryWidth"
equation "d444 = BatteryHeight"
equation "d445 = BatteryThickness"
equation "d492 = USBCReceptacleCutoutWidth"
equation "d493 = USBCReceptacleCutoutHeight"
equation "d497 = USBCReceptacleCutoutRadius"
equation "d498 = USBCReceptacleCutoutRadius"
equation "d499 = USBCReceptacleCutoutRadius"
equation "d502 = EnclosureMfgTol"
equation "d505 = -USBCReceptacleY"
equation "USBCReceptacleHeight = 8.94 mm"
equation "USBCReceptacleTolerance = 0.2 mm"
equation "EnclosureMfgTol = 0.1 mm"
equation "FrontplateThickness = 4.3 mm"
equation "LensThreadDepth = 9.2 mm" comment "Lens threaded region length + lens back focal length (BFL)"
equation "LensProtrusionInsideThickness = 13.0287 mm + 2 mm"
equation "d540 = -MountPointDepth"
equation "d542 = -MountPointDepth"
equation "d544 = LensProtrusionDepth"
equation "d546 = LensProtrusionDepth"
equation "d554 = LensProtrusionInsideThickness"
equation "d555 = LensProtrusionOutsideThickness"
equation "BackplateDovetailAngle = 10 deg"
equation "d575 = LensOringOutsideDiameter"
equation "LensOringOutsideDiameter = 13.5 mm + 0.1 mm"
equation "LensOringThickness = 1 mm"
equation "LensOringSeatDepth = 0.5 mm"
equation "d590 = MountPointDepth"
equation "d592 = MountPointDepth"
equation "d594 = LensProtrusionBoardGap"
equation "d596 = -MountPointDepth"
equation "LensProtrusionBoardGap = 0.25 mm" comment "Gap between inside lens protrusion and board"
equation "d598 = -MountPointDepth + LensProtrusionBoardGap"
equation "d599 = LensOringSeatDepth"
equation "d601 = -MountPointDepth"
equation "d602 = LensProtrusionBoardGap"
equation "d604 = MountPointHoleDepth"
equation "d611 = -MountPointDepth"
equation "MountPointHoleDepth = 5 mm"
equation "DovetailAngle = 10 deg"
equation "d616 = BoardWidth"
equation "d623 = BoardWidth"
equation "DovetailFillet = 0.5 mm"
equation "d641 = FrontplateFillet"
equation "FrontplateFillet = 2 mm"
equation "d644 = -TextEngraveDepth"
equation "TextEngraveDepth = 0.25 mm"
equation "d647 = ImageSensorX"
equation "d648 = LEDY"
equation "d649 = FrontplateThickness"
equation "d650 = LEDHoleDiameter"
equation "LEDHoleDiameter = 0.75 mm"
equation "d653 = BoardThickness"
equation "d662 = MountPointHeight"
equation "d663 = MountPoint1Width"
equation "d664 = MountPoint2Width"
equation "d665 = MountPointHeight"
equation "d666 = MountPointHeight"
equation "d667 = MountPoint3Width"
equation "d668 = MountPoint2X"
equation "d669 = MountPoint2Y"
equation "d670 = MountPoint1X"
equation "d671 = MountPoint1Y"
equation "d672 = MountPoint3Y"
equation "d673 = MountPoint3X"
equation "BackplateIndentAngle = 10 deg"
equation "BackplateIndentOffset = 17 mm"
equation "BackplateGap = 0.075 mm"
equation "BackplateIndentRadius = 1 mm"
equation "BackplateIndentWidth = 5 mm"
equation "BackplateIndentHeight = 8 mm"
equation "BackplateIndentDepth = 0.5 mm"
equation "d762 = MountPointRadius"
equation "d763 = ButtonY"
equation "d764 = ImageSensorX"
equation "ButtonY = 4.75 mm"
equation "LEDY = 28.8 mm"
equation "ButtonDiameter = 3 mm"
equation "ButtonHoleDiameter = ButtonDiameter + ButtonEnclosureClearance"
equation "d771 = FrontplateThickness"
equation "d772 = ButtonHoleDiameter"
equation "d774 = ButtonDiameter"
equation "ButtonProtrusion = 0.6 mm"
equation "ButtonHeight = MountPointDepth + FrontplateThickness + ButtonProtrusion - TactileSwitchHeight"
equation "TactileSwitchHeight = 0.6 mm + 0.1 mm"
equation "d785 = ButtonHeight"
equation "d789 = ButtonProtrusion"
equation "d790 = ButtonHoleDiameter"
equation "ButtonStopperHeight = MountPointDepth - TactileSwitchHeight"
equation "ButtonStopperDiameter = 3.6 mm"
equation "ButtonEnclosureClearance = 0.2 mm"
equation "d794 = ButtonStopperDiameter"
equation "d795 = ButtonStopperHeight"
equation "BackplateMountPointHeight = 3 mm"
equation "d809 = BackplateMountPointY"
equation "BackplateMountPointY = BoardHeight / 2"
equation "d812 = BackplateMountPointWidth"
equation "d813 = MountPointHeight"
equation "d814 = BackplateMountPointY"
equation "d815 = BackplateMountPointDepth"
equation "d819 = BackplateMountPointWidth"
equation "d820 = MountPointHeight"
equation "d821 = BackplateMountPointY"
equation "d822 = MountPointHoleDepth"
equation "d825 = BackplateHoleOffset"
equation "d826 = BackplateHoleOffset"
equation "MountPoint1Width = 3 mm"
equation "MountPoint2Width = 3 mm"
equation "MountPoint3Width = 5 mm"
equation "d857 = EnclosureThickness"
equation "d858 = BackplateThickness"
equation "d860 = BackplateThickness"
equation "d862 = BackplateThickness"
named bodies: "Body", "Front", "USBCPlugCutout", "BackplateMountPoint1", "BackplateMountPoint2"
